Autodesk Fusion 360 part; units mm, degrees
(part 9 of 15)
  spline S158 degree 5 poles (53.3841, -96.657) (53.3938, -96.6611) (53.42, -96.6723) (53.4627, -96.6904) (53.5219, -96.7153) (53.5978, -96.7469) (53.6807, -96.7809) (53.7638, -96.8145) (53.8471, -96.8478) (53.9306, -96.8808) (54.0144, -96.9134) (54.0983, -96.9457) (54.1824, -96.9776) (54.2668, -97.0092) (54.3513, -97.0405) (54.436, -97.0715) (54.5209, -97.1021) (54.606, -97.1325) (54.6913, -97.1625) (54.7768, -97.1922) (54.8624, -97.2216) (54.9483, -97.2507) (55.0342, -97.2795) (55.1204, -97.3079) (55.2067, -97.3361) (55.2932, -97.364) (55.3799, -97.3916) (55.4667, -97.4189) (55.5537, -97.4459) (55.6409, -97.4726) (55.7282, -97.499) (55.8157, -97.5252) (55.9033, -97.551) (55.991, -97.5766) (56.079, -97.6019) (56.167, -97.6269) (56.2553, -97.6516) (56.3436, -97.6761) (56.4321, -97.7003) (56.5208, -97.7242) (56.6096, -97.7478) (56.6985, -97.7712) (56.7876, -97.7943) (56.859, -97.8126) (56.9126, -97.8261) (56.9483, -97.8351) (56.9662, -97.8396) knots 0.405839 0.405839 0.405839 0.405839 0.405839 0.405839 0.414286 0.428571 0.442857 0.457143 0.471429 0.485714 0.5 0.514286 0.528571 0.542857 0.557143 0.571429 0.585714 0.6 0.614286 0.628571 0.642857 0.657143 0.671429 0.685714 0.7 0.714286 0.728571 0.742857 0.757143 0.771429 0.785714 0.8 0.814286 0.828571 0.842857 0.857143 0.871429 0.885714 0.9 0.914286 0.928571 0.942857 0.957143 0.971429 0.985714 1 1 1 1 1 1
  arc A159 (56.9662, -97.8396) -> (57.7589, -96.7807) centre (-2.0032, -52.8695) ccw
  spline S159 degree 5 poles (57.7589, -96.7807) (57.7496, -96.7648) (57.7309, -96.733) (57.7027, -96.6854) (57.6651, -96.6221) (57.6179, -96.5431) (57.5704, -96.4644) (57.5227, -96.3858) (57.4748, -96.3075) (57.4266, -96.2294) (57.3783, -96.1515) (57.3297, -96.0738) (57.2809, -95.9964) (57.2318, -95.9191) (57.1826, -95.8421) (57.1331, -95.7653) (57.0833, -95.6888) (57.0334, -95.6124) (56.9832, -95.5363) (56.9328, -95.4605) (56.8821, -95.3849) (56.8313, -95.3095) (56.7801, -95.2343) (56.7288, -95.1594) (56.6772, -95.0848) (56.6253, -95.0104) (56.5732, -94.9362) (56.5209, -94.8623) (56.4683, -94.7887) (56.4155, -94.7153) (56.3624, -94.6422) (56.3091, -94.5694) (56.2555, -94.4968) (56.2017, -94.4245) (56.1476, -94.3525) (56.0932, -94.2808) (56.0386, -94.2093) (55.9837, -94.1382) (55.9285, -94.0673) (55.8731, -93.9968) (55.8174, -93.9265) (55.7614, -93.8566) (55.7098, -93.7926) (55.6692, -93.7428) (55.6398, -93.707) (55.6217, -93.685) (55.615, -93.6769) knots -1 -1 -1 -1 -1 -1 -0.985714 -0.971429 -0.957143 -0.942857 -0.928571 -0.914286 -0.9 -0.885714 -0.871429 -0.857143 -0.842857 -0.828571 -0.814286 -0.8 -0.785714 -0.771429 -0.757143 -0.742857 -0.728571 -0.714286 -0.7 -0.685714 -0.671429 -0.657143 -0.642857 -0.628571 -0.614286 -0.6 -0.585714 -0.571429 -0.557143 -0.542857 -0.528571 -0.514286 -0.5 -0.485714 -0.471429 -0.457143 -0.442857 -0.428571 -0.414286 -0.405839 -0.405839 -0.405839 -0.405839 -0.405839 -0.405839
  arc A160 (55.615, -93.6769) -> (56.3668, -92.5941) centre (-2.0032, -52.8695) ccw
  spline S160 degree 5 poles (56.3668, -92.5941) (56.3768, -92.5976) (56.4037, -92.6069) (56.4475, -92.6219) (56.5083, -92.6425) (56.5863, -92.6685) (56.6714, -92.6965) (56.7567, -92.7242) (56.8422, -92.7515) (56.9278, -92.7784) (57.0137, -92.8049) (57.0997, -92.8311) (57.1859, -92.857) (57.2723, -92.8825) (57.3589, -92.9077) (57.4456, -92.9325) (57.5325, -92.9571) (57.6195, -92.9812) (57.7067, -93.0051) (57.7941, -93.0286) (57.8816, -93.0518) (57.9693, -93.0747) (58.0571, -93.0973) (58.1451, -93.1196) (58.2332, -93.1415) (58.3215, -93.1632) (58.4099, -93.1845) (58.4984, -93.2055) (58.5871, -93.2263) (58.676, -93.2467) (58.7649, -93.2668) (58.854, -93.2866) (58.9433, -93.3062) (59.0327, -93.3254) (59.1222, -93.3444) (59.2118, -93.363) (59.3016, -93.3814) (59.3914, -93.3995) (59.4815, -93.4173) (59.5716, -93.4348) (59.6618, -93.4521) (59.7522, -93.4691) (59.8427, -93.4857) (59.9152, -93.4989) (59.9696, -93.5086) (60.0059, -93.515) (60.0241, -93.5182) knots 0.405839 0.405839 0.405839 0.405839 0.405839 0.405839 0.414286 0.428571 0.442857 0.457143 0.471429 0.485714 0.5 0.514286 0.528571 0.542857 0.557143 0.571429 0.585714 0.6 0.614286 0.628571 0.642857 0.657143 0.671429 0.685714 0.7 0.714286 0.728571 0.742857 0.757143 0.771429 0.785714 0.8 0.814286 0.828571 0.842857 0.857143 0.871429 0.885714 0.9 0.914286 0.928571 0.942857 0.957143 0.971429 0.985714 1 1 1 1 1 1
  arc A161 (60.0241, -93.5182) -> (60.7392, -92.4054) centre (-2.0032, -52.8695) ccw
  spline S161 degree 5 poles (60.7392, -92.4054) (60.7288, -92.3902) (60.7079, -92.3599) (60.6764, -92.3144) (60.6344, -92.2539) (60.5816, -92.1785) (60.5286, -92.1034) (60.4754, -92.0284) (60.4221, -91.9537) (60.3685, -91.8792) (60.3147, -91.805) (60.2607, -91.731) (60.2065, -91.6572) (60.152, -91.5837) (60.0974, -91.5103) (60.0425, -91.4373) (59.9875, -91.3645) (59.9322, -91.2919) (59.8767, -91.2196) (59.821, -91.1475) (59.7651, -91.0757) (59.709, -91.0041) (59.6526, -90.9328) (59.5961, -90.8618) (59.5393, -90.791) (59.4822, -90.7205) (59.425, -90.6503) (59.3675, -90.5803) (59.3098, -90.5106) (59.2519, -90.4412) (59.1937, -90.372) (59.1354, -90.3032) (59.0767, -90.2346) (59.0179, -90.1664) (58.9588, -90.0984) (58.8994, -90.0307) (58.8399, -89.9634) (58.78, -89.8963) (58.72, -89.8296) (58.6596, -89.7631) (58.5991, -89.697) (58.5383, -89.6313) (58.4822, -89.5712) (58.4381, -89.5244) (58.4063, -89.4907) (58.3867, -89.4701) (58.3794, -89.4625) knots -1 -1 -1 -1 -1 -1 -0.985714 -0.971429 -0.957143 -0.942857 -0.928571 -0.914286 -0.9 -0.885714 -0.871429 -0.857143 -0.842857 -0.828571 -0.814286 -0.8 -0.785714 -0.771429 -0.757143 -0.742857 -0.728571 -0.714286 -0.7 -0.685714 -0.671429 -0.657143 -0.642857 -0.628571 -0.614286 -0.6 -0.585714 -0.571429 -0.557143 -0.542857 -0.528571 -0.514286 -0.5 -0.485714 -0.471429 -0.457143 -0.442857 -0.428571 -0.414286 -0.405839 -0.405839 -0.405839 -0.405839 -0.405839 -0.405839
  arc A162 (58.3794, -89.4625) -> (59.052, -88.3289) centre (-2.0032, -52.8695) ccw
  spline S162 degree 5 poles (59.052, -88.3289) (59.0622, -88.3316) (59.0897, -88.3389) (59.1345, -88.3508) (59.1966, -88.367) (59.2763, -88.3874) (59.3631, -88.4093) (59.4502, -88.4307) (59.5374, -88.4519) (59.6248, -88.4726) (59.7123, -88.493) (59.8, -88.513) (59.8878, -88.5326) (59.9758, -88.5519) (60.0639, -88.5709) (60.1522, -88.5894) (60.2406, -88.6077) (60.3291, -88.6256) (60.4178, -88.6432) (60.5066, -88.6604) (60.5956, -88.6773) (60.6847, -88.6939) (60.7739, -88.7102) (60.8632, -88.7261) (60.9527, -88.7417) (61.0423, -88.757) (61.132, -88.772) (61.2218, -88.7866) (61.3118, -88.801) (61.4018, -88.815) (61.492, -88.8287) (61.5823, -88.8422) (61.6727, -88.8553) (61.7632, -88.8681) (61.8539, -88.8806) (61.9446, -88.8928) (62.0354, -88.9048) (62.1264, -88.9164) (62.2174, -88.9277) (62.3086, -88.9388) (62.3999, -88.9496) (62.4912, -88.96) (62.5827, -88.9702) (62.6559, -88.9781) (62.7109, -88.9839) (62.7476, -88.9878) (62.7659, -88.9897) knots 0.405839 0.405839 0.405839 0.405839 0.405839 0.405839 0.414286 0.428571 0.442857 0.457143 0.471429 0.485714 0.5 0.514286 0.528571 0.542857 0.557143 0.571429 0.585714 0.6 0.614286 0.628571 0.642857 0.657143 0.671429 0.685714 0.7 0.714286 0.728571 0.742857 0.757143 0.771429 0.785714 0.8 0.814286 0.828571 0.842857 0.857143 0.871429 0.885714 0.9 0.914286 0.928571 0.942857 0.957143 0.971429 0.985714 1 1 1 1 1 1
  arc A163 (62.7659, -88.9897) -> (63.3998, -87.8287) centre (-2.0032, -52.8695) ccw
  spline S163 degree 5 poles (63.3998, -87.8287) (63.3883, -87.8143) (63.3653, -87.7855) (63.3307, -87.7424) (63.2844, -87.6851) (63.2264, -87.6136) (63.1682, -87.5424) (63.1098, -87.4715) (63.0512, -87.4008) (62.9925, -87.3303) (62.9335, -87.2601) (62.8744, -87.1901) (62.815, -87.1204) (62.7555, -87.0509) (62.6958, -86.9817) (62.6359, -86.9127) (62.5757, -86.844) (62.5154, -86.7756) (62.4549, -86.7074) (62.3942, -86.6395) (62.3333, -86.5718) (62.2722, -86.5045) (62.2109, -86.4374) (62.1494, -86.3705) (62.0877, -86.304) (62.0258, -86.2377) (61.9637, -86.1718) (61.9014, -86.1061) (61.8389, -86.0407) (61.7762, -85.9756) (61.7132, -85.9108) (61.6501, -85.8462) (61.5867, -85.782) (61.5231, -85.7181) (61.4593, -85.6546) (61.3953, -85.5913) (61.3311, -85.5284) (61.2666, -85.4657) (61.202, -85.4035) (61.137, -85.3415) (61.0719, -85.2799) (61.0066, -85.2186) (60.9463, -85.1627) (60.8991, -85.1191) (60.8649, -85.0879) (60.8439, -85.0687) (60.836, -85.0616) knots -1 -1 -1 -1 -1 -1 -0.985714 -0.971429 -0.957143 -0.942857 -0.928571 -0.914286 -0.9 -0.885714 -0.871429 -0.857143 -0.842857 -0.828571 -0.814286 -0.8 -0.785714 -0.771429 -0.757143 -0.742857 -0.728571 -0.714286 -0.7 -0.685714 -0.671429 -0.657143 -0.642857 -0.628571 -0.614286 -0.6 -0.585714 -0.571429 -0.557143 -0.542857 -0.528571 -0.514286 -0.5 -0.485714 -0.471429 -0.457143 -0.442857 -0.428571 -0.414286 -0.405839 -0.405839 -0.405839 -0.405839 -0.405839 -0.405839
  arc A164 (60.836, -85.0616) -> (61.4261, -83.8829) centre (-2.0032, -52.8695) ccw
  spline S164 degree 5 poles (61.4261, -83.8829) (61.4364, -83.8849) (61.4644, -83.8902) (61.5099, -83.8988) (61.5731, -83.9106) (61.654, -83.9253) (61.7422, -83.9409) (61.8305, -83.9561) (61.919, -83.9709) (62.0076, -83.9854) (62.0964, -83.9995) (62.1853, -84.0132) (62.2743, -84.0265) (62.3634, -84.0395) (62.4527, -84.0521) (62.542, -84.0643) (62.6315, -84.0762) (62.7211, -84.0878) (62.8108, -84.099) (62.9007, -84.1098) (62.9906, -84.1203) (63.0806, -84.1305) (63.1708, -84.1404) (63.261, -84.1499) (63.3514, -84.1591) (63.4418, -84.1679) (63.5324, -84.1765) (63.623, -84.1847) (63.7138, -84.1926) (63.8046, -84.2002) (63.8955, -84.2074) (63.9866, -84.2144) (64.0777, -84.221) (64.1689, -84.2273) (64.2602, -84.2334) (64.3515, -84.2391) (64.443, -84.2445) (64.5346, -84.2496) (64.6262, -84.2544) (64.7179, -84.2589) (64.8097, -84.2632) (64.9016, -84.2671) (64.9935, -84.2707) (65.0671, -84.2734) (65.1224, -84.2753) (65.1592, -84.2765) (65.1777, -84.2771) knots 0.405839 0.405839 0.405839 0.405839 0.405839 0.405839 0.414286 0.428571 0.442857 0.457143 0.471429 0.485714 0.5 0.514286 0.528571 0.542857 0.557143 0.571429 0.585714 0.6 0.614286 0.628571 0.642857 0.657143 0.671429 0.685714 0.7 0.714286 0.728571 0.742857 0.757143 0.771429 0.785714 0.8 0.814286 0.828571 0.842857 0.857143 0.871429 0.885714 0.9 0.914286 0.928571 0.942857 0.957143 0.971429 0.985714 1 1 1 1 1 1
  arc A165 (65.1777, -84.2771) -> (65.7272, -83.0738) centre (-2.0032, -52.8695) ccw
  spline S165 degree 5 poles (65.7272, -83.0738) (65.7147, -83.0603) (65.6896, -83.0332) (65.652, -82.9927) (65.6018, -82.9388) (65.5388, -82.8717) (65.4757, -82.8048) (65.4124, -82.7382) (65.3489, -82.6719) (65.2853, -82.6058) (65.2215, -82.5399) (65.1575, -82.4743) (65.0933, -82.409) (65.029, -82.344) (64.9645, -82.2792) (64.8998, -82.2147) (64.8349, -82.1505) (64.7699, -82.0865) (64.7047, -82.0228) (64.6393, -81.9594) (64.5737, -81.8963) (64.508, -81.8334) (64.442, -81.7709) (64.3759, -81.7086) (64.3096, -81.6466) (64.2432, -81.5849) (64.1765, -81.5236) (64.1097, -81.4625) (64.0426, -81.4017) (63.9754, -81.3412) (63.908, -81.2811) (63.8404, -81.2213) (63.7726, -81.1617) (63.7047, -81.1025) (63.6365, -81.0437) (63.5681, -80.9851) (63.4996, -80.9269) (63.4308, -80.8691) (63.3619, -80.8116) (63.2927, -80.7544) (63.2233, -80.6976) (63.1538, -80.6411) (63.0897, -80.5896) (63.0395, -80.5496) (63.0031, -80.5208) (62.9808, -80.5032) (62.9725, -80.4967) knots -1 -1 -1 -1 -1 -1 -0.985714 -0.971429 -0.957143 -0.942857 -0.928571 -0.914286 -0.9 -0.885714 -0.871429 -0.857143 -0.842857 -0.828571 -0.814286 -0.8 -0.785714 -0.771429 -0.757143 -0.742857 -0.728571 -0.714286 -0.7 -0.685714 -0.671429 -0.657143 -0.642857 -0.628571 -0.614286 -0.6 -0.585714 -0.571429 -0.557143 -0.542857 -0.528571 -0.514286 -0.5 -0.485714 -0.471429 -0.457143 -0.442857 -0.428571 -0.414286 -0.405839 -0.405839 -0.405839 -0.405839 -0.405839 -0.405839
  arc A166 (62.9725, -80.4967) -> (63.4769, -79.2789) centre (-2.0032, -52.8695) ccw
  spline S166 degree 5 poles (63.4769, -79.2789) (63.4874, -79.2801) (63.5157, -79.2835) (63.5617, -79.2888) (63.6255, -79.296) (63.7073, -79.3049) (63.7964, -79.3142) (63.8856, -79.3231) (63.9749, -79.3315) (64.0643, -79.3396) (64.1539, -79.3473) (64.2435, -79.3547) (64.3332, -79.3616) (64.4231, -79.3682) (64.513, -79.3744) (64.603, -79.3802) (64.6931, -79.3857) (64.7833, -79.3908) (64.8736, -79.3956) (64.964, -79.4) (65.0544, -79.4041) (65.1449, -79.4079) (65.2356, -79.4112) (65.3263, -79.4143) (65.417, -79.417) (65.5079, -79.4194) (65.5988, -79.4214) (65.6898, -79.4232) (65.7809, -79.4246) (65.872, -79.4257) (65.9633, -79.4264) (66.0545, -79.4268) (66.1459, -79.427) (66.2373, -79.4268) (66.3288, -79.4263) (66.4204, -79.4255) (66.512, -79.4243) (66.6037, -79.4229) (66.6954, -79.4212) (66.7872, -79.4191) (66.8791, -79.4168) (66.971, -79.4142) (67.0629, -79.4112) (67.1366, -79.4086) (67.1918, -79.4066) (67.2287, -79.4051) (67.2471, -79.4044) knots 0.405839 0.405839 0.405839 0.405839 0.405839 0.405839 0.414286 0.428571 0.442857 0.457143 0.471429 0.485714 0.5 0.514286 0.528571 0.542857 0.557143 0.571429 0.585714 0.6 0.614286 0.628571 0.642857 0.657143 0.671429 0.685714 0.7 0.714286 0.728571 0.742857 0.757143 0.771429 0.785714 0.8 0.814286 0.828571 0.842857 0.857143 0.871429 0.885714 0.9 0.914286 0.928571 0.942857 0.957143 0.971429 0.985714 1 1 1 1 1 1
  arc A167 (67.2471, -79.4044) -> (67.7093, -78.165) centre (-2.0032, -52.8695) ccw
  spline S167 degree 5 poles (67.7093, -78.165) (67.6959, -78.1524) (67.669, -78.1272) (67.6286, -78.0894) (67.5747, -78.0393) (67.5071, -77.9768) (67.4393, -77.9146) (67.3714, -77.8527) (67.3034, -77.7911) (67.2352, -77.7297) (67.1668, -77.6686) (67.0983, -77.6077) (67.0297, -77.5472) (66.9609, -77.4869) (66.8919, -77.4269) (66.8228, -77.3671) (66.7535, -77.3077) (66.6841, -77.2485) (66.6145, -77.1896) (66.5447, -77.131) (66.4748, -77.0728) (66.4048, -77.0148) (66.3345, -76.9571) (66.2642, -76.8997) (66.1936, -76.8426) (66.1229, -76.7858) (66.052, -76.7293) (65.981, -76.6732) (65.9098, -76.6174) (65.8385, -76.5618) (65.7669, -76.5066) (65.6953, -76.4518) (65.6234, -76.3973) (65.5514, -76.3431) (65.4792, -76.2892) (65.4068, -76.2357) (65.3343, -76.1825) (65.2616, -76.1297) (65.1887, -76.0773) (65.1156, -76.0252) (65.0424, -75.9735) (64.969, -75.9221) (64.9014, -75.8753) (64.8484, -75.839) (64.8101, -75.8129) (64.7866, -75.7969) (64.7778, -75.791) knots -1 -1 -1 -1 -1 -1 -0.985714 -0.971429 -0.957143 -0.942857 -0.928571 -0.914286 -0.9 -0.885714 -0.871429 -0.857143 -0.842857 -0.828571 -0.814286 -0.8 -0.785714 -0.771429 -0.757143 -0.742857 -0.728571 -0.714286 -0.7 -0.685714 -0.671429 -0.657143 -0.642857 -0.628571 -0.614286 -0.6 -0.585714 -0.571429 -0.557143 -0.542857 -0.528571 -0.514286 -0.5 -0.485714 -0.471429 -0.457143 -0.442857 -0.428571 -0.414286 -0.405839 -0.405839 -0.405839 -0.405839 -0.405839 -0.405839
  arc A168 (64.7778, -75.791) -> (65.1941, -74.5403) centre (-2.0032, -52.8695) ccw
  spline S168 degree 5 poles (65.1941, -74.5403) (65.2047, -74.5408) (65.2331, -74.5421) (65.2794, -74.5441) (65.3436, -74.5468) (65.4257, -74.5498) (65.5153, -74.5527) (65.6049, -74.5552) (65.6946, -74.5573) (65.7844, -74.559) (65.8742, -74.5603) (65.9641, -74.5612) (66.0541, -74.5617) (66.1442, -74.5619) (66.2343, -74.5616) (66.3246, -74.5611) (66.4148, -74.5601) (66.5052, -74.5588) (66.5955, -74.5571) (66.686, -74.5551) (66.7765, -74.5527) (66.8671, -74.5499) (66.9577, -74.5469) (67.0484, -74.5434) (67.1391, -74.5397) (67.2299, -74.5356) (67.3208, -74.5311) (67.4117, -74.5264) (67.5026, -74.5213) (67.5936, -74.5158) (67.6846, -74.5101) (67.7757, -74.504) (67.8669, -74.4976) (67.958, -74.4909) (68.0493, -74.4839) (68.1405, -74.4765) (68.2318, -74.4689) (68.3232, -74.4609) (68.4145, -74.4526) (68.506, -74.444) (68.5974, -74.4352) (68.6889, -74.426) (68.7804, -74.4165) (68.8537, -74.4087) (68.9087, -74.4026) (68.9453, -74.3986) (68.9636, -74.3965) knots 0.405839 0.405839 0.405839 0.405839 0.405839 0.405839 0.414286 0.428571 0.442857 0.457143 0.471429 0.485714 0.5 0.514286 0.528571 0.542857 0.557143 0.571429 0.585714 0.6 0.614286 0.628571 0.642857 0.657143 0.671429 0.685714 0.7 0.714286 0.728571 0.742857 0.757143 0.771429 0.785714 0.8 0.814286 0.828571 0.842857 0.857143 0.871429 0.885714 0.9 0.914286 0.928571 0.942857 0.957143 0.971429 0.985714 1 1 1 1 1 1
  arc A169 (68.9636, -74.3965) -> (69.3363, -73.1273) centre (-2.0032, -52.8695) ccw
  spline S169 degree 5 poles (69.3363, -73.1273) (69.322, -73.1157) (69.2934, -73.0925) (69.2504, -73.0577) (69.193, -73.0115) (69.1211, -72.9541) (69.0491, -72.8969) (68.977, -72.8399) (68.9047, -72.7833) (68.8323, -72.7269) (68.7598, -72.6709) (68.6871, -72.615) (68.6143, -72.5595) (68.5413, -72.5043) (68.4683, -72.4494) (68.3951, -72.3947) (68.3217, -72.3404) (68.2482, -72.2863) (68.1746, -72.2325) (68.1009, -72.1791) (68.027, -72.1259) (67.953, -72.0731) (67.8788, -72.0205) (67.8045, -71.9683) (67.7301, -71.9164) (67.6555, -71.8648) (67.5808, -71.8135) (67.5059, -71.7626) (67.4309, -71.712) (67.3558, -71.6617) (67.2805, -71.6118) (67.2051, -71.5621) (67.1295, -71.5129) (67.0538, -71.464) (66.978, -71.4154) (66.902, -71.3672) (66.8258, -71.3193) (66.7496, -71.2718) (66.6731, -71.2247) (66.5965, -71.178) (66.5198, -71.1316) (66.4429, -71.0856) (66.3721, -71.0438) (66.3167, -71.0113) (66.2767, -70.988) (66.252, -70.9737) (66.2429, -70.9684) knots -1 -1 -1 -1 -1 -1 -0.985714 -0.971429 -0.957143 -0.942857 -0.928571 -0.914286 -0.9 -0.885714 -0.871429 -0.857143 -0.842857 -0.828571 -0.814286 -0.8 -0.785714 -0.771429 -0.757143 -0.742857 -0.728571 -0.714286 -0.7 -0.685714 -0.671429 -0.657143 -0.642857 -0.628571 -0.614286 -0.6 -0.585714 -0.571429 -0.557143 -0.542857 -0.528571 -0.514286 -0.5 -0.485714 -0.471429 -0.457143 -0.442857 -0.428571 -0.414286 -0.405839 -0.405839 -0.405839 -0.405839 -0.405839 -0.405839
  arc A170 (66.2429, -70.9684) -> (66.5689, -69.6913) centre (-2.0032, -52.8695) ccw
  spline S170 degree 5 poles (66.5689, -69.6913) (66.5794, -69.691) (66.6079, -69.6903) (66.6542, -69.689) (66.7184, -69.6871) (66.8006, -69.6843) (66.8901, -69.6808) (66.9797, -69.6768) (67.0693, -69.6725) (67.159, -69.6678) (67.2487, -69.6627) (67.3384, -69.6572) (67.4282, -69.6513) (67.5181, -69.645) (67.608, -69.6384) (67.6979, -69.6313) (67.7879, -69.6239) (67.8779, -69.6162) (67.9679, -69.6081) (68.058, -69.5996) (68.1481, -69.5907) (68.2383, -69.5815) (68.3285, -69.572) (68.4187, -69.5621) (68.5089, -69.5519) (68.5992, -69.5413) (68.6895, -69.5304) (68.7798, -69.5192) (68.8701, -69.5076) (68.9605, -69.4957) (69.0509, -69.4835) (69.1413, -69.4709) (69.2318, -69.458) (69.3222, -69.4448) (69.4127, -69.4313) (69.5032, -69.4175) (69.5937, -69.4033) (69.6843, -69.3889) (69.7748, -69.3741) (69.8654, -69.359) (69.956, -69.3436) (70.0466, -69.3279) (70.1372, -69.3119) (70.2097, -69.2989) (70.2641, -69.289) (70.3004, -69.2823) (70.3185, -69.279) knots 0.405839 0.405839 0.405839 0.405839 0.405839 0.405839 0.414286 0.428571 0.442857 0.457143 0.471429 0.485714 0.5 0.514286 0.528571 0.542857 0.557143 0.571429 0.585714 0.6 0.614286 0.628571 0.642857 0.657143 0.671429 0.685714 0.7 0.714286 0.728571 0.742857 0.757143 0.771429 0.785714 0.8 0.814286 0.828571 0.842857 0.857143 0.871429 0.885714 0.9 0.914286 0.928571 0.942857 0.957143 0.971429 0.985714 1 1 1 1 1 1
  arc A171 (70.3185, -69.279) -> (70.5997, -67.9864) centre (-2.0032, -52.8695) ccw
  spline S171 degree 5 poles (70.5997, -67.9864) (70.5846, -67.9758) (70.5544, -67.9547) (70.509, -67.9231) (70.4485, -67.8811) (70.3727, -67.8289) (70.2968, -67.777) (70.2208, -67.7254) (70.1447, -67.6741) (70.0684, -67.623) (69.9921, -67.5722) (69.9156, -67.5218) (69.839, -67.4716) (69.7623, -67.4217) (69.6855, -67.3721) (69.6086, -67.3228) (69.5316, -67.2738) (69.4544, -67.2251) (69.3772, -67.1768) (69.2998, -67.1287) (69.2223, -67.081) (69.1447, -67.0335) (69.067, -66.9864) (68.9892, -66.9396) (68.9112, -66.8932) (68.8331, -66.847) (68.755, -66.8012) (68.6767, -66.7557) (68.5982, -66.7106) (68.5197, -66.6658) (68.4411, -66.6214) (68.3623, -66.5773) (68.2834, -66.5335) (68.2044, -66.4901) (68.1253, -66.4471) (68.046, -66.4044) (67.9667, -66.3621) (67.8872, -66.3202) (67.8076, -66.2786) (67.7279, -66.2375) (67.648, -66.1967) (67.568, -66.1563) (67.4945, -66.1196) (67.4369, -66.0912) (67.3952, -66.0708) (67.3697, -66.0583) (67.3602, -66.0537) knots -1 -1 -1 -1 -1 -1 -0.985714 -0.971429 -0.957143 -0.942857 -0.928571 -0.914286 -0.9 -0.885714 -0.871429 -0.857143 -0.842857 -0.828571 -0.814286 -0.8 -0.785714 -0.771429 -0.757143 -0.742857 -0.728571 -0.714286 -0.7 -0.685714 -0.671429 -0.657143 -0.642857 -0.628571 -0.614286 -0.6 -0.585714 -0.571429 -0.557143 -0.542857 -0.528571 -0.514286 -0.5 -0.485714 -0.471429 -0.457143 -0.442857 -0.428571 -0.414286 -0.405839 -0.405839 -0.405839 -0.405839 -0.405839 -0.405839
  arc A172 (67.3602, -66.0537) -> (67.5942, -64.7565) centre (-2.0032, -52.8695) ccw
  spline S172 degree 5 poles (67.5942, -64.7565) (67.6047, -64.7555) (67.633, -64.7528) (67.6792, -64.7482) (67.7431, -64.7417) (67.8248, -64.733) (67.9139, -64.7231) (68.0029, -64.7128) (68.092, -64.7021) (68.1811, -64.691) (68.2702, -64.6795) (68.3594, -64.6676) (68.4485, -64.6554) (68.5377, -64.6427) (68.6269, -64.6296) (68.7161, -64.6162) (68.8053, -64.6024) (68.8945, -64.5883) (68.9838, -64.5737) (69.073, -64.5588) (69.1623, -64.5436) (69.2515, -64.528) (69.3408, -64.512) (69.4301, -64.4958) (69.5194, -64.4791) (69.6086, -64.4621) (69.6979, -64.4448) (69.7872, -64.4271) (69.8765, -64.4092) (69.9658, -64.3908) (70.0551, -64.3722) (70.1444, -64.3532) (70.2337, -64.3339) (70.323, -64.3143) (70.4123, -64.2943) (70.5016, -64.2741) (70.5908, -64.2535) (70.6801, -64.2326) (70.7694, -64.2114) (70.8587, -64.1899) (70.9479, -64.1681) (71.0372, -64.146) (71.1264, -64.1236) (71.1978, -64.1054) (71.2514, -64.0917) (71.2871, -64.0824) (71.3049, -64.0778) knots 0.405839 0.405839 0.405839 0.405839 0.405839 0.405839 0.414286 0.428571 0.442857 0.457143 0.471429 0.485714 0.5 0.514286 0.528571 0.542857 0.557143 0.571429 0.585714 0.6 0.614286 0.628571 0.642857 0.657143 0.671429 0.685714 0.7 0.714286 0.728571 0.742857 0.757143 0.771429 0.785714 0.8 0.814286 0.828571 0.842857 0.857143 0.871429 0.885714 0.9 0.914286 0.928571 0.942857 0.957143 0.971429 0.985714 1 1 1 1 1 1
  arc A173 (71.3049, -64.0778) -> (71.4932, -62.7685) centre (-2.0032, -52.8695) ccw
  spline S173 degree 5 poles (71.4932, -62.7685) (71.4773, -62.759) (71.4457, -62.7401) (71.3982, -62.7118) (71.3348, -62.6742) (71.2555, -62.6276) (71.1761, -62.5812) (71.0966, -62.5351) (71.017, -62.4894) (70.9373, -62.4439) (70.8575, -62.3987) (70.7776, -62.3538) (70.6977, -62.3092) (70.6176, -62.2649) (70.5375, -62.2209) (70.4572, -62.1773) (70.3769, -62.1339) (70.2965, -62.0908) (70.216, -62.0481) (70.1354, -62.0057) (70.0547, -61.9636) (69.9739, -61.9218) (69.893, -61.8804) (69.812, -61.8392) (69.731, -61.7985) (69.6498, -61.758) (69.5686, -61.7179) (69.4872, -61.6781) (69.4058, -61.6387) (69.3242, -61.5996) (69.2426, -61.5609) (69.1609, -61.5225) (69.0791, -61.4845) (68.9972, -61.4469) (68.9152, -61.4096) (68.8331, -61.3727) (68.7509, -61.3361) (68.6687, -61.3) (68.5863, -61.2642) (68.5038, -61.2289) (68.4213, -61.1939) (68.3386, -61.1593) (68.2627, -61.128) (68.2032, -61.1037) (68.1602, -61.0863) (68.1338, -61.0757) (68.124, -61.0718) knots -1 -1 -1 -1 -1 -1 -0.985714 -0.971429 -0.957143 -0.942857 -0.928571 -0.914286 -0.9 -0.885714 -0.871429 -0.857143 -0.842857 -0.828571 -0.814286 -0.8 -0.785714 -0.771429 -0.757143 -0.742857 -0.728571 -0.714286 -0.7 -0.685714 -0.671429 -0.657143 -0.642857 -0.628571 -0.614286 -0.6 -0.585714 -0.571429 -0.557143 -0.542857 -0.528571 -0.514286 -0.5 -0.485714 -0.471429 -0.457143 -0.442857 -0.428571 -0.414286 -0.405839 -0.405839 -0.405839 -0.405839 -0.405839 -0.405839
  arc A174 (68.124, -61.0718) -> (68.2649, -59.7612) centre (-2.0032, -52.8695) ccw
  spline S174 degree 5 poles (68.2649, -59.7612) (68.2753, -59.7595) (68.3034, -59.7547) (68.349, -59.7469) (68.4123, -59.7358) (68.4932, -59.7213) (68.5814, -59.7051) (68.6695, -59.6885) (68.7576, -59.6715) (68.8456, -59.654) (68.9337, -59.6362) (69.0218, -59.618) (69.1098, -59.5994) (69.1979, -59.5804) (69.2859, -59.561) (69.3739, -59.5412) (69.4619, -59.5211) (69.5499, -59.5006) (69.6379, -59.4798) (69.7258, -59.4585) (69.8138, -59.437) (69.9017, -59.415) (69.9896, -59.3928) (70.0775, -59.3701) (70.1653, -59.3472) (70.2532, -59.3239) (70.341, -59.3002) (70.4288, -59.2762) (70.5166, -59.2519) (70.6044, -59.2273) (70.6921, -59.2023) (70.7798, -59.177) (70.8675, -59.1514) (70.9552, -59.1254) (71.0428, -59.0992) (71.1304, -59.0726) (71.218, -59.0457) (71.3056, -59.0185) (71.3931, -58.991) (71.4806, -58.9632) (71.5681, -58.9351) (71.6555, -58.9066) (71.743, -58.8779) (71.8129, -58.8547) (71.8653, -58.8371) (71.9002, -58.8254) (71.9177, -58.8195) knots 0.405839 0.405839 0.405839 0.405839 0.405839 0.405839 0.414286 0.428571 0.442857 0.457143 0.471429 0.485714 0.5 0.514286 0.528571 0.542857 0.557143 0.571429 0.585714 0.6 0.614286 0.628571 0.642857 0.657143 0.671429 0.685714 0.7 0.714286 0.728571 0.742857 0.757143 0.771429 0.785714 0.8 0.814286 0.828571 0.842857 0.857143 0.871429 0.885714 0.9 0.914286 0.928571 0.942857 0.957143 0.971429 0.985714 1 1 1 1 1 1
  arc A175 (71.9177, -58.8195) -> (72.0121, -57.5001) centre (-2.0032, -52.8695) ccw
  spline S175 degree 5 poles (72.0121, -57.5001) (71.9956, -57.4918) (71.9627, -57.4751) (71.9133, -57.4503) (71.8474, -57.4174) (71.765, -57.3765) (71.6825, -57.3359) (71.5999, -57.2956) (71.5172, -57.2556) (71.4345, -57.216) (71.3517, -57.1766) (71.2688, -57.1375) (71.1859, -57.0987) (71.1029, -57.0603) (71.0198, -57.0221) (70.9366, -56.9843) (70.8534, -56.9467) (70.7701, -56.9095) (70.6868, -56.8727) (70.6033, -56.8361) (70.5198, -56.7999) (70.4363, -56.764) (70.3526, -56.7284) (70.2689, -56.6931) (70.1852, -56.6582) (70.1013, -56.6237) (70.0174, -56.5895) (69.9335, -56.5556) (69.8494, -56.5221) (69.7653, -56.4889) (69.6811, -56.4561) (69.5969, -56.4237) (69.5126, -56.3916) (69.4282, -56.3599) (69.3438, -56.3285) (69.2593, -56.2976) (69.1747, -56.267) (69.09, -56.2368) (69.0053, -56.207) (68.9206, -56.1777) (68.8357, -56.1487) (68.7508, -56.1201) (68.6728, -56.0942) (68.6117, -56.0743) (68.5676, -56.06) (68.5405, -56.0513) (68.5305, -56.0481) knots -1 -1 -1 -1 -1 -1 -0.985714 -0.971429 -0.957143 -0.942857 -0.928571 -0.914286 -0.9 -0.885714 -0.871429 -0.857143 -0.842857 -0.828571 -0.814286 -0.8 -0.785714 -0.771429 -0.757143 -0.742857 -0.728571 -0.714286 -0.7 -0.685714 -0.671429 -0.657143 -0.642857 -0.628571 -0.614286 -0.6 -0.585714 -0.571429 -0.557143 -0.542857 -0.528571 -0.514286 -0.5 -0.485714 -0.471429 -0.457143 -0.442857 -0.428571 -0.414286 -0.405839 -0.405839 -0.405839 -0.405839 -0.405839 -0.405839
  circle A176 centre (-2.0032, -52.8695) radius 10.3
  circle A177 centre (-2.0032, -52.8695) radius 85
  dimension "d134" = 170
  constraint concentric A0 A177
  measures "d134" diameter of A177
extrude "Extrude1'''''" add sketch "Sketch1 (3)" against normal blind 30 separate body contours A177 makes body 11 in component "Base2"
sketch "Sketch2 (2)" plane through (0, 203.8907, 0) normal (0, 1, 0) x (-1, 0, 0) in component "Base2"
  spline S0 degree 5 poles (-72.0121, -57.5001) (-71.9956, -57.4918) (-71.9627, -57.4751) (-71.9133, -57.4503) (-71.8474, -57.4174) (-71.765, -57.3765) (-71.6825, -57.3359) (-71.5999, -57.2956) (-71.5172, -57.2556) (-71.4345, -57.216) (-71.3517, -57.1766) (-71.2688, -57.1375) (-71.1859, -57.0987) (-71.1029, -57.0603) (-71.0198, -57.0221) (-70.9366, -56.9843) (-70.8534, -56.9467) (-70.7701, -56.9095) (-70.6868, -56.8727) (-70.6033, -56.8361) (-70.5198, -56.7999) (-70.4363, -56.764) (-70.3526, -56.7284) (-70.2689, -56.6931) (-70.1852, -56.6582) (-70.1013, -56.6237) (-70.0174, -56.5895) (-69.9335, -56.5556) (-69.8494, -56.5221) (-69.7653, -56.4889) (-69.6811, -56.4561) (-69.5969, -56.4237) (-69.5126, -56.3916) (-69.4282, -56.3599) (-69.3438, -56.3285) (-69.2593, -56.2976) (-69.1747, -56.267) (-69.09, -56.2368) (-69.0053, -56.207) (-68.9206, -56.1777) (-68.8357, -56.1487) (-68.7508, -56.1201) (-68.6728, -56.0942) (-68.6117, -56.0743) (-68.5676, -56.06) (-68.5405, -56.0513) (-68.5305, -56.0481) knots -1 -1 -1 -1 -1 -1 -0.985714 -0.971429 -0.957143 -0.942857 -0.928571 -0.914286 -0.9 -0.885714 -0.871429 -0.857143 -0.842857 -0.828571 -0.814286 -0.8 -0.785714 -0.771429 -0.757143 -0.742857 -0.728571 -0.714286 -0.7 -0.685714 -0.671429 -0.657143 -0.642857 -0.628571 -0.614286 -0.6 -0.585714 -0.571429 -0.557143 -0.542857 -0.528571 -0.514286 -0.5 -0.485714 -0.471429 -0.457143 -0.442857 -0.428571 -0.414286 -0.405839 -0.405839 -0.405839 -0.405839 -0.405839 -0.405839
  arc A0 (-68.5775, -54.7308) -> (-68.5305, -56.0481) centre (2.0032, -52.8695) ccw
  spline S1 degree 5 poles (-68.5775, -54.7308) (-68.5878, -54.7283) (-68.6154, -54.7216) (-68.6604, -54.7105) (-68.7228, -54.6949) (-68.8024, -54.6747) (-68.8892, -54.6522) (-68.9759, -54.6294) (-69.0625, -54.6061) (-69.1491, -54.5824) (-69.2357, -54.5584) (-69.3222, -54.5339) (-69.4087, -54.5091) (-69.4952, -54.4838) (-69.5816, -54.4582) (-69.668, -54.4322) (-69.7544, -54.4059) (-69.8407, -54.3792) (-69.9269, -54.3521) (-70.0131, -54.3247) (-70.0993, -54.2969) (-70.1854, -54.2687) (-70.2715, -54.2402) (-70.3576, -54.2114) (-70.4436, -54.1822) (-70.5295, -54.1527) (-70.6155, -54.1228) (-70.7013, -54.0927) (-70.7871, -54.0621) (-70.8729, -54.0313) (-70.9587, -54.0001) (-71.0443, -53.9686) (-71.13, -53.9368) (-71.2156, -53.9047) (-71.3011, -53.8723) (-71.3866, -53.8395) (-71.4721, -53.8064) (-71.5574, -53.7731) (-71.6428, -53.7394) (-71.7281, -53.7054) (-71.8133, -53.6711) (-71.8985, -53.6365) (-71.9837, -53.6016) (-72.0518, -53.5735) (-72.1028, -53.5522) (-72.1368, -53.538) (-72.1538, -53.5309) knots 0.405839 0.405839 0.405839 0.405839 0.405839 0.405839 0.414286 0.428571 0.442857 0.457143 0.471429 0.485714 0.5 0.514286 0.528571 0.542857 0.557143 0.571429 0.585714 0.6 0.614286 0.628571 0.642857 0.657143 0.671429 0.685714 0.7 0.714286 0.728571 0.742857 0.757143 0.771429 0.785714 0.8 0.814286 0.828571 0.842857 0.857143 0.871429 0.885714 0.9 0.914286 0.928571 0.942857 0.957143 0.971429 0.985714 1 1 1 1 1 1
  arc A1 (-72.1538, -52.2081) -> (-72.1538, -53.5309) centre (2.0032, -52.8695) ccw
  spline S2 degree 5 poles (-72.1538, -52.2081) (-72.1368, -52.201) (-72.1028, -52.1867) (-72.0518, -52.1655) (-71.9837, -52.1373) (-71.8985, -52.1025) (-71.8133, -52.0679) (-71.7281, -52.0336) (-71.6428, -51.9996) (-71.5574, -51.9659) (-71.4721, -51.9325) (-71.3866, -51.8995) (-71.3011, -51.8667) (-71.2156, -51.8343) (-71.13, -51.8021) (-71.0443, -51.7703) (-70.9587, -51.7388) (-70.8729, -51.7077) (-70.7871, -51.6768) (-70.7013, -51.6463) (-70.6155, -51.6161) (-70.5295, -51.5863) (-70.4436, -51.5567) (-70.3576, -51.5276) (-70.2715, -51.4987) (-70.1854, -51.4702) (-70.0993, -51.4421) (-70.0131, -51.4143) (-69.9269, -51.3869) (-69.8407, -51.3598) (-69.7544, -51.3331) (-69.668, -51.3067) (-69.5816, -51.2807) (-69.4952, -51.2551) (-69.4087, -51.2299) (-69.3222, -51.2051) (-69.2357, -51.1806) (-69.1491, -51.1565) (-69.0625, -51.1329) (-68.9759, -51.1096) (-68.8892, -51.0867) (-68.8024, -51.0643) (-68.7228, -51.044) (-68.6604, -51.0285) (-68.6154, -51.0174) (-68.5878, -51.0107) (-68.5775, -51.0082) knots -1 -1 -1 -1 -1 -1 -0.985714 -0.971429 -0.957143 -0.942857 -0.928571 -0.914286 -0.9 -0.885714 -0.871429 -0.857143 -0.842857 -0.828571 -0.814286 -0.8 -0.785714 -0.771429 -0.757143 -0.742857 -0.728571 -0.714286 -0.7 -0.685714 -0.671429 -0.657143 -0.642857 -0.628571 -0.614286 -0.6 -0.585714 -0.571429 -0.557143 -0.542857 -0.528571 -0.514286 -0.5 -0.485714 -0.471429 -0.457143 -0.442857 -0.428571 -0.414286 -0.405839 -0.405839 -0.405839 -0.405839 -0.405839 -0.405839
  arc A2 (-68.5305, -49.6909) -> (-68.5775, -51.0082) centre (2.0032, -52.8695) ccw
  spline S3 degree 5 poles (-68.5305, -49.6909) (-68.5405, -49.6877) (-68.5676, -49.679) (-68.6117, -49.6647) (-68.6728, -49.6447) (-68.7508, -49.6189) (-68.8357, -49.5903) (-68.9206, -49.5613) (-69.0053, -49.5319) (-69.09, -49.5021) (-69.1747, -49.4719) (-69.2593, -49.4414) (-69.3438, -49.4104) (-69.4282, -49.3791) (-69.5126, -49.3474) (-69.5969, -49.3153) (-69.6811, -49.2828) (-69.7653, -49.25) (-69.8494, -49.2169) (-69.9335, -49.1834) (-70.0174, -49.1495) (-70.1013, -49.1153) (-70.1852, -49.0807) (-70.2689, -49.0458) (-70.3526, -49.0106) (-70.4363, -48.975) (-70.5198, -48.9391) (-70.6033, -48.9029) (-70.6868, -48.8663) (-70.7701, -48.8294) (-70.8534, -48.7922) (-70.9366, -48.7547) (-71.0198, -48.7169) (-71.1029, -48.6787) (-71.1859, -48.6402) (-71.2688, -48.6015) (-71.3517, -48.5624) (-71.4345, -48.523) (-71.5172, -48.4833) (-71.5999, -48.4433) (-71.6825, -48.403) (-71.765, -48.3625) (-71.8474, -48.3216) (-71.9133, -48.2887) (-71.9627, -48.2638) (-71.9956, -48.2472) (-72.0121, -48.2389) knots 0.405839 0.405839 0.405839 0.405839 0.405839 0.405839 0.414286 0.428571 0.442857 0.457143 0.471429 0.485714 0.5 0.514286 0.528571 0.542857 0.557143 0.571429 0.585714 0.6 0.614286 0.628571 0.642857 0.657143 0.671429 0.685714 0.7 0.714286 0.728571 0.742857 0.757143 0.771429 0.785714 0.8 0.814286 0.828571 0.842857 0.857143 0.871429 0.885714 0.9 0.914286 0.928571 0.942857 0.957143 0.971429 0.985714 1 1 1 1 1 1
  arc A3 (-71.9177, -46.9195) -> (-72.0121, -48.2389) centre (2.0032, -52.8695) ccw
  spline S4 degree 5 poles (-71.9177, -46.9195) (-71.9002, -46.9136) (-71.8653, -46.9018) (-71.8129, -46.8843) (-71.743, -46.861) (-71.6555, -46.8323) (-71.5681, -46.8039) (-71.4806, -46.7758) (-71.3931, -46.748) (-71.3056, -46.7204) (-71.218, -46.6932) (-71.1304, -46.6664) (-71.0428, -46.6398) (-70.9552, -46.6135) (-70.8675, -46.5876) (-70.7798, -46.562) (-70.6921, -46.5367) (-70.6044, -46.5117) (-70.5166, -46.487) (-70.4288, -46.4627) (-70.341, -46.4387) (-70.2532, -46.4151) (-70.1653, -46.3918) (-70.0775, -46.3688) (-69.9896, -46.3462) (-69.9017, -46.3239) (-69.8138, -46.302) (-69.7258, -46.2804) (-69.6379, -46.2592) (-69.5499, -46.2384) (-69.4619, -46.2179) (-69.3739, -46.1977) (-69.2859, -46.178) (-69.1979, -46.1586) (-69.1098, -46.1396) (-69.0218, -46.121) (-68.9337, -46.1028) (-68.8456, -46.0849) (-68.7576, -46.0675) (-68.6695, -46.0505) (-68.5814, -46.0339) (-68.4932, -46.0177) (-68.4123, -46.0032) (-68.349, -45.9921) (-68.3034, -45.9842) (-68.2753, -45.9795) (-68.2649, -45.9777) knots -1 -1 -1 -1 -1 -1 -0.985714 -0.971429 -0.957143 -0.942857 -0.928571 -0.914286 -0.9 -0.885714 -0.871429 -0.857143 -0.842857 -0.828571 -0.814286 -0.8 -0.785714 -0.771429 -0.757143 -0.742857 -0.728571 -0.714286 -0.7 -0.685714 -0.671429 -0.657143 -0.642857 -0.628571 -0.614286 -0.6 -0.585714 -0.571429 -0.557143 -0.542857 -0.528571 -0.514286 -0.5 -0.485714 -0.471429 -0.457143 -0.442857 -0.428571 -0.414286 -0.405839 -0.405839 -0.405839 -0.405839 -0.405839 -0.405839
  arc A4 (-68.124, -44.6672) -> (-68.2649, -45.9777) centre (2.0032, -52.8695) ccw
  spline S5 degree 5 poles (-68.124, -44.6672) (-68.1338, -44.6632) (-68.1602, -44.6526) (-68.2032, -44.6353) (-68.2627, -44.611) (-68.3386, -44.5796) (-68.4213, -44.5451) (-68.5038, -44.5101) (-68.5863, -44.4747) (-68.6687, -44.439) (-68.7509, -44.4028) (-68.8331, -44.3663) (-68.9152, -44.3294) (-68.9972, -44.2921) (-69.0791, -44.2545) (-69.1609, -44.2165) (-69.2426, -44.1781) (-69.3242, -44.1394) (-69.4058, -44.1003) (-69.4872, -44.0608) (-69.5686, -44.0211) (-69.6498, -43.981) (-69.731, -43.9405) (-69.812, -43.8997) (-69.893, -43.8586) (-69.9739, -43.8172) (-70.0547, -43.7754) (-70.1354, -43.7333) (-70.216, -43.6909) (-70.2965, -43.6481) (-70.3769, -43.6051) (-70.4572, -43.5617) (-70.5375, -43.518) (-70.6176, -43.4741) (-70.6977, -43.4298) (-70.7776, -43.3852) (-70.8575, -43.3403) (-70.9373, -43.2951) (-71.017, -43.2496) (-71.0966, -43.2038) (-71.1761, -43.1577) (-71.2555, -43.1114) (-71.3348, -43.0647) (-71.3982, -43.0272) (-71.4457, -42.9989) (-71.4773, -42.98) (-71.4932, -42.9705) knots 0.405839 0.405839 0.405839 0.405839 0.405839 0.405839 0.414286 0.428571 0.442857 0.457143 0.471429 0.485714 0.5 0.514286 0.528571 0.542857 0.557143 0.571429 0.585714 0.6 0.614286 0.628571 0.642857 0.657143 0.671429 0.685714 0.7 0.714286 0.728571 0.742857 0.757143 0.771429 0.785714 0.8 0.814286 0.828571 0.842857 0.857143 0.871429 0.885714 0.9 0.914286 0.928571 0.942857 0.957143 0.971429 0.985714 1 1 1 1 1 1
  arc A5 (-71.3049, -41.6612) -> (-71.4932, -42.9705) centre (2.0032, -52.8695) ccw
  spline S6 degree 5 poles (-71.3049, -41.6612) (-71.2871, -41.6565) (-71.2514, -41.6473) (-71.1978, -41.6335) (-71.1264, -41.6154) (-71.0372, -41.5929) (-70.9479, -41.5708) (-70.8587, -41.549) (-70.7694, -41.5275) (-70.6801, -41.5063) (-70.5908, -41.4854) (-70.5016, -41.4649) (-70.4123, -41.4446) (-70.323, -41.4247) (-70.2337, -41.4051) (-70.1444, -41.3858) (-70.0551, -41.3668) (-69.9658, -41.3481) (-69.8765, -41.3298) (-69.7872, -41.3118) (-69.6979, -41.2942) (-69.6086, -41.2768) (-69.5194, -41.2599) (-69.4301, -41.2432) (-69.3408, -41.2269) (-69.2515, -41.211) (-69.1623, -41.1954) (-69.073, -41.1801) (-68.9838, -41.1652) (-68.8945, -41.1507) (-68.8053, -41.1365) (-68.7161, -41.1227) (-68.6269, -41.1093) (-68.5377, -41.0963) (-68.4485, -41.0836) (-68.3594, -41.0713) (-68.2702, -41.0594) (-68.1811, -41.0479) (-68.092, -41.0368) (-68.0029, -41.0261) (-67.9139, -41.0158) (-67.8248, -41.006) (-67.7431, -40.9973) (-67.6792, -40.9907) (-67.633, -40.9862) (-67.6047, -40.9834) (-67.5942, -40.9824) knots -1 -1 -1 -1 -1 -1 -0.985714 -0.971429 -0.957143 -0.942857 -0.928571 -0.914286 -0.9 -0.885714 -0.871429 -0.857143 -0.842857 -0.828571 -0.814286 -0.8 -0.785714 -0.771429 -0.757143 -0.742857 -0.728571 -0.714286 -0.7 -0.685714 -0.671429 -0.657143 -0.642857 -0.628571 -0.614286 -0.6 -0.585714 -0.571429 -0.557143 -0.542857 -0.528571 -0.514286 -0.5 -0.485714 -0.471429 -0.457143 -0.442857 -0.428571 -0.414286 -0.405839 -0.405839 -0.405839 -0.405839 -0.405839 -0.405839
  arc A6 (-67.3602, -39.6853) -> (-67.5942, -40.9824) centre (2.0032, -52.8695) ccw
  spline S7 degree 5 poles (-67.3602, -39.6853) (-67.3697, -39.6806) (-67.3952, -39.6682) (-67.4369, -39.6478) (-67.4945, -39.6193) (-67.568, -39.5826) (-67.648, -39.5422) (-67.7279, -39.5015) (-67.8076, -39.4603) (-67.8872, -39.4188) (-67.9667, -39.3769) (-68.046, -39.3346) (-68.1253, -39.2919) (-68.2044, -39.2489) (-68.2834, -39.2055) (-68.3623, -39.1617) (-68.4411, -39.1176) (-68.5197, -39.0732) (-68.5982, -39.0284) (-68.6767, -38.9832) (-68.755, -38.9377) (-68.8331, -38.8919) (-68.9112, -38.8458) (-68.9892, -38.7993) (-69.067, -38.7525) (-69.1447, -38.7054) (-69.2223, -38.658) (-69.2998, -38.6102) (-69.3772, -38.5622) (-69.4544, -38.5138) (-69.5316, -38.4651) (-69.6086, -38.4162) (-69.6855, -38.3669) (-69.7623, -38.3173) (-69.839, -38.2674) (-69.9156, -38.2172) (-69.9921, -38.1667) (-70.0684, -38.116) (-70.1447, -38.0649) (-70.2208, -38.0136) (-70.2968, -37.9619) (-70.3727, -37.91) (-70.4485, -37.8578) (-70.509, -37.8159) (-70.5544, -37.7842) (-70.5846, -37.7631) (-70.5997, -37.7525) knots 0.405839 0.405839 0.405839 0.405839 0.405839 0.405839 0.414286 0.428571 0.442857 0.457143 0.471429 0.485714 0.5 0.514286 0.528571 0.542857 0.557143 0.571429 0.585714 0.6 0.614286 0.628571 0.642857 0.657143 0.671429 0.685714 0.7 0.714286 0.728571 0.742857 0.757143 0.771429 0.785714 0.8 0.814286 0.828571 0.842857 0.857143 0.871429 0.885714 0.9 0.914286 0.928571 0.942857 0.957143 0.971429 0.985714 1 1 1 1 1 1
  arc A7 (-70.3185, -36.46) -> (-70.5997, -37.7525) centre (2.0032, -52.8695) ccw
  spline S8 degree 5 poles (-70.3185, -36.46) (-70.3004, -36.4566) (-70.2641, -36.45) (-70.2097, -36.4401) (-70.1372, -36.427) (-70.0466, -36.411) (-69.956, -36.3953) (-69.8654, -36.38) (-69.7748, -36.3649) (-69.6843, -36.3501) (-69.5937, -36.3356) (-69.5032, -36.3215) (-69.4127, -36.3077) (-69.3222, -36.2941) (-69.2318, -36.2809) (-69.1413, -36.2681) (-69.0509, -36.2555) (-68.9605, -36.2433) (-68.8701, -36.2314) (-68.7798, -36.2198) (-68.6895, -36.2085) (-68.5992, -36.1976) (-68.5089, -36.1871) (-68.4187, -36.1768) (-68.3285, -36.167) (-68.2383, -36.1574) (-68.1481, -36.1482) (-68.058, -36.1394) (-67.9679, -36.1309) (-67.8779, -36.1228) (-67.7879, -36.115) (-67.6979, -36.1076) (-67.608, -36.1006) (-67.5181, -36.0939) (-67.4282, -36.0877) (-67.3384, -36.0818) (-67.2487, -36.0763) (-67.159, -36.0712) (-67.0693, -36.0664) (-66.9797, -36.0621) (-66.8901, -36.0582) (-66.8006, -36.0547) (-66.7184, -36.0519) (-66.6542, -36.0499) (-66.6079, -36.0487) (-66.5794, -36.0479) (-66.5689, -36.0477) knots -1 -1 -1 -1 -1 -1 -0.985714 -0.971429 -0.957143 -0.942857 -0.928571 -0.914286 -0.9 -0.885714 -0.871429 -0.857143 -0.842857 -0.828571 -0.814286 -0.8 -0.785714 -0.771429 -0.757143 -0.742857 -0.728571 -0.714286 -0.7 -0.685714 -0.671429 -0.657143 -0.642857 -0.628571 -0.614286 -0.6 -0.585714 -0.571429 -0.557143 -0.542857 -0.528571 -0.514286 -0.5 -0.485714 -0.471429 -0.457143 -0.442857 -0.428571 -0.414286 -0.405839 -0.405839 -0.405839 -0.405839 -0.405839 -0.405839
  arc A8 (-66.2429, -34.7705) -> (-66.5689, -36.0477) centre (2.0032, -52.8695) ccw
  spline S9 degree 5 poles (-66.2429, -34.7705) (-66.252, -34.7652) (-66.2767, -34.751) (-66.3167, -34.7277) (-66.3721, -34.6952) (-66.4429, -34.6533) (-66.5198, -34.6073) (-66.5965, -34.561) (-66.6731, -34.5142) (-66.7496, -34.4671) (-66.8258, -34.4196) (-66.902, -34.3718) (-66.978, -34.3236) (-67.0538, -34.275) (-67.1295, -34.2261) (-67.2051, -34.1768) (-67.2805, -34.1272) (-67.3558, -34.0773) (-67.4309, -34.027) (-67.5059, -33.9764) (-67.5808, -33.9254) (-67.6555, -33.8741) (-67.7301, -33.8226) (-67.8045, -33.7706) (-67.8788, -33.7184) (-67.953, -33.6659) (-68.027, -33.613) (-68.1009, -33.5599) (-68.1746, -33.5064) (-68.2482, -33.4527) (-68.3217, -33.3986) (-68.3951, -33.3442) (-68.4683, -33.2896) (-68.5413, -33.2347) (-68.6143, -33.1794) (-68.6871, -33.1239) (-68.7598, -33.0681) (-68.8323, -33.012) (-68.9047, -32.9557) (-68.977, -32.899) (-69.0491, -32.8421) (-69.1211, -32.7849) (-69.193, -32.7274) (-69.2504, -32.6812) (-69.2934, -32.6465) (-69.322, -32.6233) (-69.3363, -32.6116) knots 0.405839 0.405839 0.405839 0.405839 0.405839 0.405839 0.414286 0.428571 0.442857 0.457143 0.471429 0.485714 0.5 0.514286 0.528571 0.542857 0.557143 0.571429 0.585714 0.6 0.614286 0.628571 0.642857 0.657143 0.671429 0.685714 0.7 0.714286 0.728571 0.742857 0.757143 0.771429 0.785714 0.8 0.814286 0.828571 0.842857 0.857143 0.871429 0.885714 0.9 0.914286 0.928571 0.942857 0.957143 0.971429 0.985714 1 1 1 1 1 1
  arc A9 (-68.9636, -31.3424) -> (-69.3363, -32.6116) centre (2.0032, -52.8695) ccw
  spline S10 degree 5 poles (-68.9636, -31.3424) (-68.9453, -31.3404) (-68.9087, -31.3363) (-68.8537, -31.3303) (-68.7804, -31.3225) (-68.6889, -31.313) (-68.5974, -31.3038) (-68.506, -31.2949) (-68.4145, -31.2863) (-68.3232, -31.2781) (-68.2318, -31.2701) (-68.1405, -31.2624) (-68.0493, -31.2551) (-67.958, -31.2481) (-67.8669, -31.2414) (-67.7757, -31.235) (-67.6846, -31.2289) (-67.5936, -31.2231) (-67.5026, -31.2177) (-67.4117, -31.2126) (-67.3208, -31.2078) (-67.2299, -31.2034) (-67.1391, -31.1993) (-67.0484, -31.1955) (-66.9577, -31.1921) (-66.8671, -31.189) (-66.7765, -31.1863) (-66.686, -31.1839) (-66.5955, -31.1819) (-66.5052, -31.1802) (-66.4148, -31.1789) (-66.3246, -31.1779) (-66.2343, -31.1773) (-66.1442, -31.1771) (-66.0541, -31.1772) (-65.9641, -31.1778) (-65.8742, -31.1787) (-65.7844, -31.18) (-65.6946, -31.1817) (-65.6049, -31.1838) (-65.5153, -31.1862) (-65.4257, -31.1891) (-65.3436, -31.1922) (-65.2794, -31.1948) (-65.2331, -31.1969) (-65.2047, -31.1982) (-65.1941, -31.1987) knots -1 -1 -1 -1 -1 -1 -0.985714 -0.971429 -0.957143 -0.942857 -0.928571 -0.914286 -0.9 -0.885714 -0.871429 -0.857143 -0.842857 -0.828571 -0.814286 -0.8 -0.785714 -0.771429 -0.757143 -0.742857 -0.728571 -0.714286 -0.7 -0.685714 -0.671429 -0.657143 -0.642857 -0.628571 -0.614286 -0.6 -0.585714 -0.571429 -0.557143 -0.542857 -0.528571 -0.514286 -0.5 -0.485714 -0.471429 -0.457143 -0.442857 -0.428571 -0.414286 -0.405839 -0.405839 -0.405839 -0.405839 -0.405839 -0.405839
  arc A10 (-64.7778, -29.948) -> (-65.1941, -31.1987) centre (2.0032, -52.8695) ccw
  spline S11 degree 5 poles (-64.7778, -29.948) (-64.7866, -29.9421) (-64.8101, -29.9261) (-64.8484, -29.9) (-64.9014, -29.8636) (-64.969, -29.8168) (-65.0424, -29.7655) (-65.1156, -29.7138) (-65.1887, -29.6617) (-65.2616, -29.6092) (-65.3343, -29.5564) (-65.4068, -29.5033) (-65.4792, -29.4498) (-65.5514, -29.3959) (-65.6234, -29.3417) (-65.6953, -29.2872) (-65.7669, -29.2323) (-65.8385, -29.1771) (-65.9098, -29.1216) (-65.981, -29.0658) (-66.052, -29.0096) (-66.1229, -28.9531) (-66.1936, -28.8964) (-66.2642, -28.8393) (-66.3345, -28.7819) (-66.4048, -28.7242) (-66.4748, -28.6662) (-66.5447, -28.6079) (-66.6145, -28.5493) (-66.6841, -28.4905) (-66.7535, -28.4313) (-66.8228, -28.3718) (-66.8919, -28.3121) (-66.9609, -28.2521) (-67.0297, -28.1918) (-67.0983, -28.1312) (-67.1668, -28.0704) (-67.2352, -28.0093) (-67.3034, -27.9479) (-67.3714, -27.8862) (-67.4393, -27.8243) (-67.5071, -27.7621) (-67.5747, -27.6997) (-67.6286, -27.6495) (-67.669, -27.6118) (-67.6959, -27.5866) (-67.7093, -27.5739) knots 0.405839 0.405839 0.405839 0.405839 0.405839 0.405839 0.414286 0.428571 0.442857 0.457143 0.471429 0.485714 0.5 0.514286 0.528571 0.542857 0.557143 0.571429 0.585714 0.6 0.614286 0.628571 0.642857 0.657143 0.671429 0.685714 0.7 0.714286 0.728571 0.742857 0.757143 0.771429 0.785714 0.8 0.814286 0.828571 0.842857 0.857143 0.871429 0.885714 0.9 0.914286 0.928571 0.942857 0.957143 0.971429 0.985714 1 1 1 1 1 1
  arc A11 (-67.2471, -26.3346) -> (-67.7093, -27.5739) centre (2.0032, -52.8695) ccw
  spline S12 degree 5 poles (-67.2471, -26.3346) (-67.2287, -26.3338) (-67.1918, -26.3324) (-67.1366, -26.3303) (-67.0629, -26.3277) (-66.971, -26.3248) (-66.8791, -26.3222) (-66.7872, -26.3198) (-66.6954, -26.3178) (-66.6037, -26.3161) (-66.512, -26.3146) (-66.4204, -26.3135) (-66.3288, -26.3127) (-66.2373, -26.3122) (-66.1459, -26.312) (-66.0545, -26.3121) (-65.9633, -26.3126) (-65.872, -26.3133) (-65.7809, -26.3144) (-65.6898, -26.3158) (-65.5988, -26.3175) (-65.5079, -26.3196) (-65.417, -26.322) (-65.3263, -26.3247) (-65.2356, -26.3277) (-65.1449, -26.3311) (-65.0544, -26.3348) (-64.964, -26.3389) (-64.8736, -26.3433) (-64.7833, -26.3481) (-64.6931, -26.3532) (-64.603, -26.3587) (-64.513, -26.3646) (-64.4231, -26.3708) (-64.3332, -26.3774) (-64.2435, -26.3843) (-64.1539, -26.3916) (-64.0643, -26.3993) (-63.9749, -26.4074) (-63.8856, -26.4159) (-63.7964, -26.4248) (-63.7073, -26.4341) (-63.6255, -26.4429) (-63.5617, -26.4502) (-63.5157, -26.4555) (-63.4874, -26.4588) (-63.4769, -26.4601) knots -1 -1 -1 -1 -1 -1 -0.985714 -0.971429 -0.957143 -0.942857 -0.928571 -0.914286 -0.9 -0.885714 -0.871429 -0.857143 -0.842857 -0.828571 -0.814286 -0.8 -0.785714 -0.771429 -0.757143 -0.742857 -0.728571 -0.714286 -0.7 -0.685714 -0.671429 -0.657143 -0.642857 -0.628571 -0.614286 -0.6 -0.585714 -0.571429 -0.557143 -0.542857 -0.528571 -0.514286 -0.5 -0.485714 -0.471429 -0.457143 -0.442857 -0.428571 -0.414286 -0.405839 -0.405839 -0.405839 -0.405839 -0.405839 -0.405839
  arc A12 (-62.9725, -25.2423) -> (-63.4769, -26.4601) centre (2.0032, -52.8695) ccw
  spline S13 degree 5 poles (-62.9725, -25.2423) (-62.9808, -25.2358) (-63.0031, -25.2181) (-63.0395, -25.1894) (-63.0897, -25.1493) (-63.1538, -25.0978) (-63.2233, -25.0414) (-63.2927, -24.9846) (-63.3619, -24.9274) (-63.4308, -24.8699) (-63.4996, -24.812) (-63.5681, -24.7538) (-63.6365, -24.6953) (-63.7047, -24.6364) (-63.7726, -24.5772) (-63.8404, -24.5177) (-63.908, -24.4579) (-63.9754, -24.3977) (-64.0426, -24.3373) (-64.1097, -24.2765) (-64.1765, -24.2154) (-64.2432, -24.154) (-64.3096, -24.0923) (-64.3759, -24.0304) (-64.442, -23.9681) (-64.508, -23.9055) (-64.5737, -23.8427) (-64.6393, -23.7796) (-64.7047, -23.7162) (-64.7699, -23.6525) (-64.8349, -23.5885) (-64.8998, -23.5243) (-64.9645, -23.4598) (-65.029, -23.395) (-65.0933, -23.3299) (-65.1575, -23.2646) (-65.2215, -23.199) (-65.2853, -23.1332) (-65.3489, -23.0671) (-65.4124, -23.0008) (-65.4757, -22.9341) (-65.5388, -22.8673) (-65.6018, -22.8002) (-65.652, -22.7463) (-65.6896, -22.7058) (-65.7147, -22.6787) (-65.7272, -22.6651) knots 0.405839 0.405839 0.405839 0.405839 0.405839 0.405839 0.414286 0.428571 0.442857 0.457143 0.471429 0.485714 0.5 0.514286 0.528571 0.542857 0.557143 0.571429 0.585714 0.6 0.614286 0.628571 0.642857 0.657143 0.671429 0.685714 0.7 0.714286 0.728571 0.742857 0.757143 0.771429 0.785714 0.8 0.814286 0.828571 0.842857 0.857143 0.871429 0.885714 0.9 0.914286 0.928571 0.942857 0.957143 0.971429 0.985714 1 1 1 1 1 1
  arc A13 (-65.1777, -21.4619) -> (-65.7272, -22.6651) centre (2.0032, -52.8695) ccw